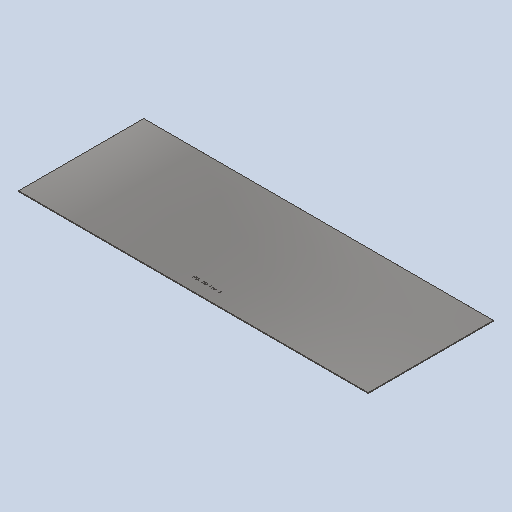
# Autodesk Inventor part: MSC 702 face 2
Saved by Autodesk Inventor 2025 (Build 290162010, 162A)
## iProperties
Created: 2024-06-16
Part Number: MSC 702 face 2
Material: Stainless Steel
Document SubType Name: Sheet Metal
Designer: admin
Density: 8 g/cm^3
Sheet Metal Rule: AISI304 3mm Die 32
Appearance: Semi-Polished
Stock Number: МОО 702 морда 3
Mass: 18825.6 g
Surface Area: 15808.6 cm^2
Volume: 2353.2 cm^3
Flat Pattern Width: 53 cm
Flat Pattern Length: 148 cm
Flat Pattern Area: 7844 cm^2
Sheet Metal Width: 530,000 mm
Sheet Metal Length: 1480,000 mm
Sheet Metal Area: 784400,000 mm^2
Author: admin
Autodesk Inventor part; units mm, degrees
ref_plane "YZ Plane" through (0, 0, 0) normal (1, 0, 0) x (0, 1, 0)
ref_plane "XZ Plane" through (0, 0, 0) normal (0, 1, 0) x (-1, 0, 0)
ref_plane "XY Plane" through (0, 0, 0) normal (0, 0, 1) x (1, 0, 0)
sketch "Sketch1" plane through (0, 0, 0) normal (0, 0, 1) x (1, 0, 0)
  line L0 (-740, 0) -> (740, 0)
  line L1 (740, 0) -> (740, -530)
  line L2 (740, -530) -> (-740, -530)
  line L3 (-740, -530) -> (-740, 0)
  point P0 (0, 0)
  point P1 (0, 0)
  dimension "d0" = 1480
  dimension "d1" = 530
  measures "d0" distance of L1.end L2.end
  measures "d1" distance of L0.end L1.end
extrude "Plate1" add sketch "Sketch1" along normal blind 3
sketch "Sketch2" plane through (0, 0, 3) normal (0, 0, 1) x (1, 0, 0)
  line L0 (-55, -480) -> (-55, -468) construction
  line L1 (-55, -468) -> (55, -468) construction
  line L2 (55, -468) -> (55, -480) construction
  line L3 (55, -480) -> (-55, -480) construction
  line L4 (740, -530) -> (-740, -530) projected
  point P0 (0, 0)
  point P1 (0, -480)
  point P2 (0, -530)
  dimension "d3" = 12
  dimension "d4" = 110
  dimension "d5" = 50
  constraints: 2 midpoint, 1 vertical alignment, 2 other
  measures "d3" distance of L1.end L2.end
  measures "d4" distance between parallel lines of L0 L2
  measures "d5" distance between parallel lines of L4 L3
mark "Mark1"
equation "\"d2\" = Thickness"
equation "\"BendReliefWidth\" = Thickness"
equation "\"BendReliefDepth\" = 0.5 * Thickness"
equation "\"CornerReliefSize\" = 4 * Thickness"
equation "\"MinimumRemnant\" = 2 * Thickness"
equation "\"TransitionRadius\" = BendRadius"
equation "\"JacobiRadiusSize\" = BendRadius"
equation "\"GapSize\" = Thickness"
equation "\"Thickness\" = 3"
equation "\"BendRadius\" = 5"
body "Solid1"
